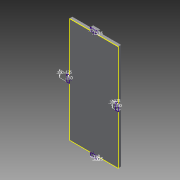
# Autodesk Inventor part: Birdhouse Wall
Saved by Autodesk Inventor 2015 (Build 190159000, 159)
## iProperties
Created: 2018-03-09
Part Number: Birdhouse Wall
Material: Generic
Document SubType Name: Modeling
Designer: Administrator
Density: 1 g/cm^3
Appearance: Default
Author: Administrator
Autodesk Inventor part; units mm, degrees
ref_plane "YZ Plane" through (0, 0, 0) normal (1, 0, 0) x (0, 1, 0)
ref_plane "XZ Plane" through (0, 0, 0) normal (0, 1, 0) x (-1, 0, 0)
ref_plane "XY Plane" through (0, 0, 0) normal (0, 0, 1) x (1, 0, 0)
sketch "Sketch1" plane through (0, 0, 0) normal (0, 0, 1) x (1, 0, 0)
  line L0 (0, 0) -> (52.9336, 0)
  line L1 (52.9336, 0) -> (52.9336, 114.3)
  line L2 (52.9336, 114.3) -> (0, 114.3)
  line L3 (0, 114.3) -> (0, 0)
  dimension "d0" = 114.3
  dimension "d1" = 52.9336
  constraints: 8 end point, 2 parallel, 1 horizontal, 1 perpendicular
  measures "d0" distance of L2.end L0.start
  measures "d1" distance of L0.start L0.end
extrude "Extrusion1" add sketch "Sketch1" along normal blind 3.175
sketch "Sketch2" plane through (0, 0, 3.175) normal (0, 0, 1) x (1, 0, 0)
  line L0 (0, 114.3) -> (0, 0) projected
  line L1 (52.9336, 0) -> (52.9336, 114.3) projected
  line L2 (0, 60.96) -> (-3.175, 60.96)
  line L3 (-3.175, 60.96) -> (-3.175, 53.34)
  line L4 (-3.175, 53.34) -> (0, 53.34)
  line L5 (0, 53.34) -> (0, 60.96)
  line L6 (52.9336, 60.96) -> (49.7586, 60.96)
  line L7 (49.7586, 60.96) -> (49.7586, 53.34)
  line L8 (49.7586, 53.34) -> (52.9336, 53.34)
  line L9 (52.9336, 53.34) -> (52.9336, 60.96)
  line L10 (52.9336, 114.3) -> (0, 114.3) projected
  line L11 (0, 0) -> (52.9336, 0) projected
  line L12 (22.6568, 114.3) -> (22.6568, 117.475)
  line L13 (22.6568, 117.475) -> (30.2768, 117.475)
  line L14 (30.2768, 117.475) -> (30.2768, 114.3)
  line L15 (30.2768, 114.3) -> (22.6568, 114.3)
  line L16 (30.2768, 0) -> (30.2768, -3.175)
  line L17 (30.2768, -3.175) -> (22.6568, -3.175)
  line L18 (22.6568, -3.175) -> (22.6568, 0)
  line L19 (22.6568, 0) -> (30.2768, 0)
  point P0 (0, 57.15)
  point P1 (52.9336, 57.15)
  point P2 (26.4668, 114.3)
  point P3 (26.4668, 0)
  dimension "d4" = 3.81
  dimension "d5" = 7.62
  dimension "d6" = 3.175
  dimension "d7" = 3.81
  dimension "d8" = 7.62
  dimension "d9" = 3.175
  dimension "d10" = 3.81
  dimension "d11" = 3.81
  dimension "d12" = 3.175
  dimension "d13" = 7.62
  dimension "d14" = 3.81
  dimension "d15" = 3.175
  constraints: 32 end point, 9 perpendicular, 8 point on line, 4 midpoint, 4 parallel, 2 collinear, 2 vertical
  measures "d4" distance from line of point (0, 57.15) L2
  measures "d5" distance between parallel lines of L2 L4
  measures "d6" distance between parallel lines of L0 L3
  measures "d7" distance from line of point (52.934, 57.15) L6
  measures "d8" distance between parallel lines of L6 L8
  measures "d9" distance between parallel lines of L1 L7
  measures "d10" distance from line of L14 point (26.467, 114.3)
  measures "d11" distance from line of L12 point (26.467, 114.3)
  measures "d12" distance between parallel lines of L10 L13
  measures "d13" distance between parallel lines of L16 L18
  measures "d14" distance from line of L16 point (26.467, 0)
  measures "d15" distance between parallel lines of L17 L11
extrude "Extrusion2" add sketch "Sketch2" against normal blind 3.175 contours L0 L4 L3 L2 | L12 L13 L14 L10 | L11 L16 L17 L18 | L1 L8 L7 L6
extrude "Extrusion3" cut sketch "Sketch2" against normal blind 3.175 contours L1 L8 L7 L6
body "Solid1"
